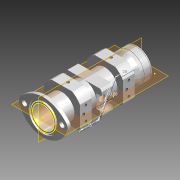
# Autodesk Inventor part: throttle_ETC
Saved by Autodesk Inventor 2015 (Build 190159000, 159)
## iProperties
Created: 2015-04-14
Part Number: throttle_ETC
Material: Aluminum 6061
Description: insert part description/title
Document SubType Name: Modeling
Designer: frank
Density: 2.7 g/cm^3
Appearance: Aluminum - Flat
Part Category: insert part category here and press enter to fill value
Author: frank
Autodesk Inventor part; units mm, degrees
ref_plane "XZ Plane" through (0, 0, 0) normal (0, 1, 0) x (-1, 0, 0)
sketch "Sketch1" plane through (0, 0, 0) normal (0, 0, 1) x (1, 0, 0)
  line L0 (14, -120) -> (14, -22.588)
  line L1 (14.382, -20.4813) -> (16.618, -14.5187)
  line L2 (17, -12.412) -> (17, -2)
  line L3 (19.0526, -13.7225) -> (16, -21.8627)
  line L4 (16, -21.8627) -> (16, -120)
  line L5 (19.5, 0) -> (19, 0)
  line L6 (16, -120) -> (14, -120)
  line L7 (19, -1) -> (19.4, -1)
  line L8 (19.4, -1) -> (19.4, 0)
  line L9 (19.4, 0) -> (19.5, 0)
  line L10 (19, -8.5) -> (19.4, -8.5)
  line L11 (19.4, -8.5) -> (19.4, -9.5)
  line L12 (19.4, -9.5) -> (19, -9.5)
  line L13 (19, -9.5) -> (19.0526, -13.7225)
  line L14 (19, -1) -> (19, -8.5)
  line L15 (0, 0) -> (0, -57.1164)
  arc A0 (19, 0) -> (17, -2) centre (19, -2) ccw
  arc A1 (16.618, -14.5187) -> (17, -12.412) centre (11, -12.412) ccw
  arc A2 (14.382, -20.4813) -> (14, -22.588) centre (20, -22.588) ccw
  point P0 (14, -21.5)
  point P1 (17, -13.5)
  point P2 (17, 0)
  point P3 (17, 0)
  point P4 (16, -38.699)
  dimension "d1" = 13.5
  dimension "d2" = 21.5
  dimension "d3" = 14
  dimension "d4" = 120
  dimension "d5" = 2
  dimension "d6" = 0.4
  dimension "d7" = 1
  dimension "d8" = 0.4
  dimension "d9" = 1
  dimension "d10" = 8.5
  dimension "d124" = 19
  dimension "d125" = 2
  dimension "d126" = 2
  dimension "d127" = 2
  dimension "d128" = 6
  constraints: 32 end point, 8 point on line, 6 point on circle, 6 tangent, 3 centre point, 3 parallel, 2 coincident, 2 horizontal, 2 perpendicular, 1 collinear, 1 equal radius, 1 vertical, 1 other
  measures "d1" distance of point (17, -13.5) point (17, 0)
  measures "d2" vertical distance of point (14, -21.5) point (17, 0)
  measures "d3" distance from line of L15.start L0
  measures "d4" vertical distance of point (17, 0) L0.start
  measures "d5" distance between parallel lines of L1 L3
  measures "d6" distance of L7.start L7.end
  measures "d7" distance of L7.end L8.end
  measures "d8" distance of L11.end L12.end
  measures "d9" distance of L10.end L11.end
  measures "d10" distance between parallel lines of L9 L10
  measures "d124" distance between parallel lines of L15 L14
  measures "d125" distance between parallel lines of L2 L14
  measures "d126" distance from line of L2 L12.end
  measures "d127" radius of A0
  measures "d128" radius of A1
revolve "Revolution1" add sketch "Sketch1" angle 360 about axis through (0, 0, 0) along (0, -1, 0)
sketch "Sketch5" plane through (0, -120, 0) normal (0, -1, 0) x (1, 0, 0)
  circle A0 centre (0, 0) radius 14 projected
  circle A1 centre (0, 0) radius 16 projected
  point P0 (-16, 0)
  constraints: 1 horizontal alignment, 1 other
sketch "Sketch7" plane through (0, -120, 0) normal (0, -1, 0) x (1, 0, 0)
  circle A0 centre (0, 0) radius 14 projected
  circle A1 centre (-24, 3.4731) radius 3.25
  circle A2 centre (24, 3.4731) radius 3.25
  circle A3 centre (0, 0) radius 18.5
  arc A4 (-29.548, 8.1402) -> (-31.0133, 1.6358) centre (-24, 3.4731) ccw
  arc A5 (-31.0133, 1.6358) -> (0, -22.5) centre (0.2614, 9.8292) ccw
  arc A6 (0, 22.5) -> (-29.548, 8.1402) centre (1.3447, -17.8473) ccw
  line L0 (-34.5214, 0) -> (40.2242, 0) construction
  circle A7 centre (0, 0) radius 14 construction
  line L1 (0, -32.9352) -> (0, 39.8381)
  arc A8 (31.0133, 1.6358) -> (29.548, 8.1402) centre (24, 3.4731) ccw
  arc A9 (0, -22.5) -> (31.0133, 1.6358) centre (-0.2614, 9.8292) ccw
  arc A10 (29.548, 8.1402) -> (0, 22.5) centre (-1.3447, -17.8473) ccw
  point P0 (0, -18.5)
  dimension "d28" = 37
  dimension "d24" = 6.5
  dimension "d25" = 48
  dimension "d26" = 7
  dimension "d27" = 6.5
  dimension "d29" = 0
  dimension "d30" = 0
  dimension "d31" = 4
  dimension "d33" = 22.5
  dimension "d34" = 4
  constraints: 12 point on circle, 8 centre point, 5 symmetric about line, 4 end point, 2 tangent, 1 horizontal, 1 vertical, 1 vertical alignment, 6 other
  measures "d24" diameter of A2
  measures "d25" distance of A2.centre A1.centre
  measures "d27" diameter of A1
  measures "d29" distance of A1.centre A4.centre
  measures "d30" distance of A1.centre A4.centre
  measures "d31" radial gap between concentric circles of A1 A4
  measures "d33" distance of A6.start point (0, 0)
  measures "d34" distance of point (0, -18.5) A5.end
extrude "Extrusion2" add sketch "Sketch7" against normal blind 4 contours A0 L1 A3 | A0 L1 A3 | L1 A10 A8 A9 A3 | A3 L1 A5 A4 A6
sketch "Sketch8" plane through (0.2614, -120, 9.8292) normal (0, -1, 0) x (0.789176, 0, -0.6141671)
  circle A0 centre (5.8304, -7.9175) radius 16
  circle A1 centre (5.8304, -7.9175) radius 18.5 projected
  circle A2 centre (5.8304, -7.9175) radius 18.5
  constraints: 2 centre point, 2 coincident, 1 concentric
extrude "Extrusion3" cut sketch "Sketch8" against normal blind 2
fillet "Fillet1" radius 2 1 edges at (-16, -116, 0)
sketch "Sketch9" plane through (0, 0, 0) normal (1, 0, 0) x (0, 1, 0)
  line L0 (-21.8627, 16) -> (-114, 16) projected
  line L1 (-21.8627, 16) -> (-21.8627, -16) projected
  line L2 (-32.5282, 0) -> (-141.2862, 0) construction
  line L3 (-53.8627, -16) -> (-67.8627, -16)
  line L4 (-67.8627, -16) -> (-67.8627, -26.5)
  line L5 (-67.8627, -26.5) -> (-53.8627, -26.5)
  line L6 (-53.8627, -26.5) -> (-53.8627, -16)
  line L7 (-80.8627, -16) -> (-95.8627, -16)
  line L8 (-95.8627, -16) -> (-95.8627, -26.5)
  line L9 (-95.8627, -26.5) -> (-80.8627, -26.5)
  line L10 (-80.8627, -26.5) -> (-80.8627, -16)
  line L11 (-21.8627, -16) -> (-114, -16) construction
  line L12 (-40.8627, -16) -> (-25.8627, -16)
  line L13 (-25.8627, -16) -> (-25.8627, -26.5)
  line L14 (-25.8627, -26.5) -> (-40.8627, -26.5)
  line L15 (-40.8627, -26.5) -> (-40.8627, -16)
  line L16 (-88.3627, -26.5) -> (-88.3627, -22.6244) construction
  line L17 (-60.8627, -26.5) -> (-60.8627, -20.6547) construction
  point P0 (0, 0)
  dimension "d42" = 14
  dimension "d47" = 10.5
  dimension "d48" = 32
  dimension "d55" = 10.5
  dimension "d57" = 35
  dimension "d58" = 20
  dimension "d59" = 20
  dimension "d60" = 35
  dimension "d61" = 10.5
  constraints: 30 end point, 6 parallel, 4 horizontal, 3 perpendicular, 2 collinear, 2 midpoint, 2 vertical, 1 point on line
  measures "d42" distance of L4.end L5.end
  measures "d47" distance of L5.end L3.start
  measures "d48" distance between parallel lines of L1 L6
  measures "d55" distance of L9.end L7.start
  measures "d57" distance between parallel lines of L8 L17
  measures "d58" distance between parallel lines of L10 L17
  measures "d59" distance between parallel lines of L15 L17
  measures "d60" distance between parallel lines of L13 L17
  measures "d61" distance of L12.end L13.end
revolve "Revolution2" add sketch "Sketch9" angle 360 about axis through (0, -32.5282, 0) along (0, -1, 0)
sketch "Sketch10" plane through (0, 0, 0) normal (1, 0, 0) x (0, 1, 0)
  line L0 (-95.8627, 16) -> (-114, 16) construction
  line L1 (-95.8627, -16) -> (-114, -16) construction
  line L2 (-53.8627, 26.5) -> (-53.8627, -26.5) construction
  line L3 (-67.8627, 26.5) -> (-67.8627, -26.5) construction
  circle A0 centre (-60.8627, 0) radius 4
  line L4 (-53.8627, -26.5) -> (-67.8627, -26.5) projected
  line L5 (-144, 0) -> (24, 0) construction
  point P0 (0, 0)
  point P1 (-60.8627, -26.5)
  dimension "d50" = 8
  constraints: 1 centre point, 1 midpoint, 1 point on line, 1 vertical alignment
  measures "d50" diameter of A0
extrude "Extrusion4" cut sketch "Sketch10" along normal through all both and the other way through all
sketch "Sketch11" plane through (0, 0, 0) normal (0, 0, 1) x (1, 0, 0)
  line L0 (-26.5, -53.8627) -> (26.5, -53.8627) construction
  line L1 (16, -53.8627) -> (-16, -53.8627) construction
  line L2 (-26.5, -53.8627) -> (26.5, -53.8627) construction
  line L3 (14, -120) -> (14, -22.588) construction
  line L4 (14, -120) -> (14, -22.588) construction
  line L5 (14, -120) -> (14, -22.588) construction
  line L6 (14, -120) -> (14, -22.588) construction
  line L7 (-14, -120) -> (-14, -22.588) construction
  line L8 (-26.5, -53.8627) -> (-26.5, -67.8627) construction
  line L9 (-26.5, -67.8627) -> (26.5, -67.8627) construction
  line L10 (27.5381, -60.9184) -> (-34.1758, -60.9184)
  line L11 (16, -40.8627) -> (16, -53.8627) construction
  line L12 (-16, -40.8627) -> (-16, -53.8627) construction
  line L13 (-16, -67.8627) -> (-16, -80.8627) construction
  line L14 (16, -67.8627) -> (16, -80.8627) construction
  line L15 (26.5, -53.8627) -> (26.5, -67.8627) construction
  line L16 (26.5, -60.8627) -> (16, -60.8627)
  line L17 (16, -60.8627) -> (16, -49.9184)
  line L18 (16, -49.9184) -> (26.5, -49.9184)
  line L19 (26.5, -49.9184) -> (26.5, -60.8627)
  line L20 (-26.5, -60.9184) -> (-16, -60.9184)
  line L21 (-16, -60.9184) -> (-16, -49.9184)
  line L22 (-16, -49.9184) -> (-26.5, -49.9184)
  line L23 (-26.5, -49.9184) -> (-26.5, -60.9184)
  point P0 (0, 0)
  dimension "d62" = 11
  constraints: 18 end point, 5 point on line, 4 parallel, 3 horizontal, 2 perpendicular, 1 midpoint
  measures "d62" distance of L22.end L20.start
revolve "Revolution3" cut sketch "Sketch11" angle 360 about axis through (27.5381, -60.9184, 0) along (-1, 0, 0)
sketch "Sketch12" plane through (0, 0, 0) normal (0, 0, 1) x (1, 0, 0)
  line L0 (-25.1204, -53.8627) -> (25.1204, -53.8627) construction
  line L1 (-25.0893, -67.8627) -> (25.0893, -67.8627) construction
  line L2 (-16, -40.8627) -> (-16, -53.8627) construction
  line L3 (-16, -67.8627) -> (-16, -80.8627) construction
  line L4 (16, -40.8627) -> (16, -53.8627) construction
  line L5 (16, -67.8627) -> (16, -80.8627) construction
  line L6 (-25.1204, -53.8627) -> (-23, -53.8627)
  line L7 (-23, -53.8627) -> (-23, -67.8627)
  line L8 (-23, -67.8627) -> (-25.1204, -67.8627)
  line L9 (-25.1204, -67.8627) -> (-25.1204, -53.8627)
  line L10 (-25.0893, -67.8627) -> (-16, -67.8627) construction
  line L11 (0, 4.0598) -> (0, -79.7186) construction
  line L12 (25.1204, -53.8627) -> (23, -53.8627)
  line L13 (23, -53.8627) -> (23, -67.8627)
  line L14 (23, -67.8627) -> (25.1204, -67.8627)
  line L15 (25.1204, -67.8627) -> (25.1204, -53.8627)
  line L16 (-26.5, -25.8627) -> (-26.5, -40.8627) construction
  line L17 (-26.5, -25.8627) -> (26.5, -25.8627) construction
  line L18 (-25.1204, -53.8627) -> (25.1204, -53.8627) construction
  line L19 (-26.5, -80.8627) -> (26.5, -80.8627) construction
  line L20 (-26.5, -95.8627) -> (26.5, -95.8627) construction
  line L21 (-26.5, -40.8627) -> (26.5, -40.8627) construction
  line L22 (-26.5, -40.8627) -> (-23, -40.8627)
  line L23 (-23, -40.8627) -> (-23, -25.8627)
  line L24 (-23, -25.8627) -> (-26.5, -25.8627)
  line L25 (-26.5, -25.8627) -> (-26.5, -40.8627)
  line L26 (-26.5, -80.8627) -> (-23, -80.8627)
  line L27 (-23, -80.8627) -> (-23, -95.8627)
  line L28 (-23, -95.8627) -> (-26.5, -95.8627)
  line L29 (-26.5, -95.8627) -> (-26.5, -80.8627)
  line L30 (-16, -21.8627) -> (-16, -25.8627) construction
  line L31 (-16, -95.8627) -> (-16, -114) construction
  line L32 (26.5, -25.8627) -> (26.5, -40.8627) construction
  line L33 (26.5, -40.8627) -> (23, -40.8627)
  line L34 (23, -40.8627) -> (23, -25.8627)
  line L35 (23, -25.8627) -> (26.5, -25.8627)
  line L36 (26.5, -25.8627) -> (26.5, -40.8627)
  line L37 (26.5, -80.8627) -> (23, -80.8627)
  line L38 (23, -80.8627) -> (23, -95.8627)
  line L39 (23, -95.8627) -> (26.5, -95.8627)
  line L40 (26.5, -95.8627) -> (26.5, -80.8627)
  point P0 (0, 0)
  point P1 (25.0893, -67.8627)
  dimension "d64" = 7
  dimension "d69" = 7
  constraints: 52 end point, 14 symmetric about line, 6 parallel, 6 point on line, 3 horizontal, 3 perpendicular, 1 vertical
  measures "d64" distance between parallel lines of L2 L7
  measures "d69" distance between parallel lines of L30 L23
extrude "Extrusion5" cut sketch "Sketch12" along normal through all both and the other way through all
sketch "Sketch13" plane through (0, 0, 0) normal (1, 0, 0) x (0, 1, 0)
  line L0 (-25.8627, 26.5) -> (-25.8627, -26.5) construction
  line L1 (-40.8627, 16) -> (-53.8627, 16) construction
  line L2 (-33.4184, 0) -> (-136.7664, 0) construction
  line L3 (-80.8627, -26.5) -> (-95.8627, -26.5) construction
  line L4 (-25.8627, -26.5) -> (-40.8627, -26.5) construction
  line L5 (-53.8627, -26.5) -> (-67.8627, -26.5) construction
  line L6 (-40.8627, -16) -> (-53.8627, -16) construction
  line L7 (-25.8627, -26.5) -> (-95.8627, -26.5)
  line L8 (-95.8627, -26.5) -> (-95.8627, -16)
  line L9 (-95.8627, -16) -> (-25.8627, -16)
  line L10 (-25.8627, -16) -> (-25.8627, -26.5)
  line L11 (-40.8627, 16) -> (-40.8627, -16) projected
  line L12 (-53.8627, 26.5) -> (-67.8627, 26.5)
  line L13 (-67.8627, 26.5) -> (-67.8627, 16)
  line L14 (-67.8627, 16) -> (-53.8627, 16)
  line L15 (-53.8627, 16) -> (-53.8627, 26.5)
  line L16 (-40.8627, 26.5) -> (-40.8627, 13.1624) projected
  line L17 (-25.8627, 26.5) -> (-40.8627, 26.5)
  line L18 (-40.8627, 26.5) -> (-40.8627, 23)
  line L19 (-40.8627, 23) -> (-25.8627, 23)
  line L20 (-25.8627, 23) -> (-25.8627, 26.5)
  line L21 (-95.8627, 26.5) -> (-95.8627, 13.1624) projected
  line L22 (-80.8627, 26.5) -> (-95.8627, 26.5)
  line L23 (-95.8627, 26.5) -> (-95.8627, 23)
  line L24 (-95.8627, 23) -> (-80.8627, 23)
  line L25 (-80.8627, 23) -> (-80.8627, 26.5)
  point P0 (0, 0)
  point P1 (-95.8627, 26.5)
  point P2 (-67.8627, 26.5)
  point P3 (-95.8627, 16)
  point P4 (-95.8627, -16)
  point P5 (-80.9184, 16)
  dimension "d113" = 7
  constraints: 42 end point, 11 symmetric about line, 6 parallel, 4 horizontal, 3 perpendicular, 3 point on line
  measures "d113" distance between parallel lines of L1 L19
extrude "Extrusion6" cut sketch "Sketch13" along normal through all both and the other way through all
sketch "Sketch14" plane through (-23, -40.8627, 13.1624) normal (-1, 0, 0) x (0, 0, 1)
  line L0 (-13.1624, 64.9184) -> (-13.1624, -103.0816) construction
  line L1 (-26.3249, 15) -> (0, 15) construction
  line L2 (0, -40) -> (0, -55) construction
  line L3 (-26.3249, -40) -> (0, -40) construction
  line L4 (-26.3249, -55) -> (-26.3249, -40) construction
  line L5 (0, -55) -> (-26.3249, -55) construction
  circle A0 centre (-22.1624, 7.5) radius 2 construction
  circle A1 centre (-22.1624, -47.5) radius 2 construction
  line L6 (-26.3249, 0) -> (-26.3249, 15) construction
  line L7 (-26.3249, -55) -> (-26.3249, -40) construction
  line L8 (-13.1624, 17.742) -> (-13.1624, -35.3687)
  circle A2 centre (-4.1624, 7.5) radius 2 construction
  circle A3 centre (-4.1624, -47.5) radius 2 construction
  point P0 (-13.1624, 40.8627)
  point P1 (-26.3249, 7.5)
  point P2 (-26.3249, -47.5)
  point P3 (-26.3249, -47.5)
  point P4 (-26.3249, 7.5)
  dimension "d86" = 4
  dimension "d87" = 4
  dimension "d88" = 9
  dimension "d89" = 9
  constraints: 4 centre point, 4 end point, 4 midpoint, 2 horizontal alignment, 2 point on line, 2 symmetric about line, 2 other
  measures "d86" diameter of A0
  measures "d87" diameter of A1
  measures "d88" distance from line of L0 A1.centre
  measures "d89" distance from line of L0 A0.centre
hole "Hole4" at (-23, -33.3627, -9) at (-23, -88.3627, -9) at (-23, -33.3627, 9) at (-23, -88.3627, 9) direction (1, 0, 0) diameter 3.459 depth 6 tip angle 118 thread size "M4x0.5" class "6H" standard "ISO Metric profile"
sketch "Sketch15" plane through (-23, -40.8627, 13.1624) normal (-1, 0, 0) x (0, 0, 1)
  circle A0 centre (-13.1624, 10.5) radius 2.25 projected
  circle A1 centre (-13.1624, -44.5) radius 2.25 projected
  point P0 (-13.1624, 40.8627)
hole "Hole5" at (-23, -30.3627, 0) at (-23, -85.3627, 0) direction (1, 0, 0) diameter 4.134 depth 7 tip angle 118 thread size "M5x0.8" class "6H" standard "ISO Metric profile"
sketch "Sketch16" plane through (23, -40.8627, -13.1624) normal (1, 0, 0) x (0, 0, -1)
  circle A0 centre (-13.1624, 4.5) radius 2.25 projected
  circle A1 centre (-13.1624, -50.5) radius 2.25 projected
  point P0 (-13.1624, 40.8627)
hole "Hole6" at (23, -36.3627, 0) at (23, -91.3627, 0) direction (-1, 0, 0) diameter 4.134 depth 7 tip angle 118 thread size "M5x0.8" class "6H" standard "ISO Metric profile"
sketch "Sketch17" plane through (23, -40.8627, -13.1624) normal (1, 0, 0) x (0, 0, -1)
  line L0 (-13.1624, -20) -> (-30.483, -10) construction
  line L1 (-13.1624, -37.5) -> (-13.1624, -2.5) construction
  line L2 (-30.483, -10) -> (-30.483, 15) construction
  line L3 (-13.1624, -20) -> (4.1581, -30) construction
  line L4 (2.8376, -55) -> (2.8376, -40) construction
  line L5 (4.1581, -30) -> (4.1581, -55) construction
  point P0 (-13.1624, 40.8627)
  dimension "d118" = 20
  dimension "d119" = 60
  dimension "d120" = 25
  dimension "d121" = 20
  dimension "d123" = 25
  constraints: 10 end point, 3 vertical, 1 collinear, 3 other
  measures "d118" distance of L0.start L0.end
  measures "d119" angle of L1 L0
  measures "d120" distance of L0.end L2.end
  measures "d121" distance of L0.start L3.end
  measures "d123" distance of L3.end L5.end
mirror "Mirror1" about plane through (0, 0, 0) normal (1, 0, 0) of "Hole4"
sketch "Sketch18" plane through (-13.1624, -40.8627, 23) normal (0, 0, 1) x (1, 0, 0)
  line L0 (0, 0) -> (0, 15) construction
  line L1 (26.3249, 0) -> (0, 0) construction
  line L2 (26.3249, 15) -> (26.3249, 0) construction
  line L3 (0, 15) -> (26.3249, 15) construction
  line L4 (0, -55) -> (0, -40) construction
  line L5 (26.3249, -55) -> (0, -55) construction
  line L6 (26.3249, -40) -> (26.3249, -55) construction
  line L7 (0, -40) -> (26.3249, -40) construction
  line L8 (13.1624, -103.1373) -> (13.1624, 64.8627) construction
  point P0 (13.1624, 40.8627)
  point P1 (13.1624, 7.5)
  point P2 (13.1624, -47.5)
  constraints: 2 point on line
hole "Hole7" at (0, -33.3627, 23) at (0, -88.3627, 23) direction (0, 0, -1) diameter 4 depth 23 tip angle 118
equation "\"d53\" = d50"
body "Solid1"
